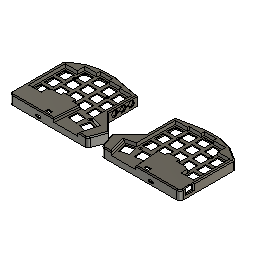
top_3x5_2 (Autodesk Fusion 360 design; units mm, degrees)
Autodesk Fusion 360 part; units mm, degrees
sketch "case_plate_3x5_2" plane through (0, 0, 0) normal (0, 0, 1) x (1, 0, 0)
  line L0 (-131.5, -112.72) -> (-13.7052, -112.72)
  line L1 (-131.5, -30.9488) -> (-131.5, -112.72)
  line L2 (-72.4047, -13.5) -> (-91.6231, -13.5)
  line L3 (-91.6231, -13.5) -> (-111.8983, -18.5688)
  line L4 (-32.5, -21.174) -> (-72.3112, -13.518)
  line L5 (-6.0652, -91.7293) -> (-32.5, -65.3353)
  line L6 (-111.8983, -18.5688) -> (-131.5, -30.9488)
  line L7 (-72.3112, -13.518) -> (-72.4047, -13.5)
  line L8 (-13.7052, -112.72) -> (-6.0652, -91.7293)
  line L9 (-32.5, -65.3353) -> (-32.5, -21.174)
  line L10 (-113.0931, -15.7752) -> (-134.5, -29.2953)
  line L11 (-72.1189, -10.5) -> (-91.9924, -10.5)
  line L12 (-29.5, -64.0913) -> (-29.5, -18.6959)
  line L13 (-11.6046, -115.72) -> (-2.5919, -90.9579)
  line L14 (-134.5, -115.72) -> (-11.6046, -115.72)
  line L15 (-2.5919, -90.9579) -> (-29.5, -64.0913)
  line L16 (-91.9924, -10.5) -> (-113.0931, -15.7752)
  line L17 (-134.5, -29.2953) -> (-134.5, -115.72)
  line L18 (-29.5, -18.6959) -> (-72.1189, -10.5)
  line L19 (-72.2904, -12.3) -> (-91.7708, -12.3)
  line L20 (-132.7, -30.2874) -> (-132.7, -113.92)
  line L21 (-4.6759, -91.4207) -> (-31.3, -64.8377)
  line L22 (-31.3, -20.1828) -> (-72.2904, -12.3)
  line L23 (-132.7, -113.92) -> (-12.865, -113.92)
  line L24 (-12.865, -113.92) -> (-4.6759, -91.4207)
  line L25 (-31.3, -64.8377) -> (-31.3, -20.1828)
  line L26 (-91.7708, -12.3) -> (-112.3762, -17.4513)
  line L27 (-112.3762, -17.4513) -> (-132.7, -30.2874)
  line L28 (-133.3, -29.9567) -> (-133.3, -114.52)
  line L29 (-12.4448, -114.52) -> (-3.9812, -91.2664)
  line L30 (-112.6152, -16.8926) -> (-133.3, -29.9567)
  line L31 (-71.9712, -11.7504) -> (-72.2332, -11.7)
  line L32 (-30.7, -64.5889) -> (-30.7, -19.6872)
  line L33 (-133.3, -114.52) -> (-12.4448, -114.52)
  line L34 (-30.7, -19.6872) -> (-71.9712, -11.7504)
  line L35 (-3.9812, -91.2664) -> (-30.7, -64.5889)
  line L36 (-72.2332, -11.7) -> (-91.8447, -11.7)
  line L37 (-91.8447, -11.7) -> (-112.6152, -16.8926)
  circle A0 centre (-108, -39.5) radius 2.2
  circle A1 centre (-56, -39.5) radius 2.2
  circle A2 centre (-39.8644, -83.3241) radius 2.2
  line L38 (-96.5, -91.61) -> (-129.5, -91.61)
  line L39 (-96.5, -109.61) -> (-96.5, -91.61)
  line L40 (-129.5, -109.61) -> (-96.5, -109.61)
  line L41 (-129.5, -91.61) -> (-129.5, -109.61)
  line L42 (-92.975, -106.99) -> (-92.975, -112.84)
  line L43 (-84.175, -112.84) -> (-84.175, -106.99)
  line L44 (-84.175, -106.99) -> (-92.975, -106.99)
  line L45 (-82.175, -107.975) -> (-82.175, -111.475)
  line L46 (-82.175, -111.475) -> (-73.175, -111.475)
  line L47 (-73.175, -107.975) -> (-82.175, -107.975)
  line L48 (-73.175, -111.475) -> (-73.175, -107.975)
  line L49 (-17.3936, -82.1718) -> (-25.1718, -74.3936)
  line L50 (-25.1718, -74.3936) -> (-31.6064, -80.8282)
  line L51 (-21.0041, -85.7823) -> (-17.3936, -82.1718)
  line L52 (-96.8, -88.45) -> (-96.8, -79.55)
  line L53 (-96.8, -79.55) -> (-105.2875, -79.55)
  line L54 (-105.4, -79.6909) -> (-105.4, -88.45)
  line L55 (-105.4, -88.45) -> (-96.8, -88.45)
  line L56 (-127, -73) -> (-127, -87)
  line L57 (-113, -73) -> (-127, -73)
  line L58 (-113, -87) -> (-113, -73)
  line L59 (-127, -87) -> (-113, -87)
  line L60 (-127, -54) -> (-127, -68)
  line L61 (-113, -68) -> (-113, -54)
  line L62 (-127, -68) -> (-113, -68)
  line L63 (-113, -54) -> (-127, -54)
  line L64 (-113, -35) -> (-127, -35)
  line L65 (-127, -35) -> (-127, -49)
  line L66 (-127, -49) -> (-113, -49)
  line L67 (-113, -49) -> (-113, -35)
  line L68 (-94, -61) -> (-108, -61)
  line L69 (-94, -75) -> (-94, -61)
  line L70 (-108, -61) -> (-108, -75)
  line L71 (-108, -75) -> (-94, -75)
  line L72 (-108, -56) -> (-94, -56)
  line L73 (-94, -56) -> (-94, -42)
  line L74 (-94, -42) -> (-108, -42)
  line L75 (-108, -42) -> (-108, -56)
  line L76 (-94, -37) -> (-94, -23)
  line L77 (-108, -37) -> (-94, -37)
  line L78 (-108, -23) -> (-108, -37)
  line L79 (-94, -23) -> (-108, -23)
  line L80 (-89, -70) -> (-75, -70)
  line L81 (-89, -56) -> (-89, -70)
  line L82 (-75, -56) -> (-89, -56)
  line L83 (-75, -70) -> (-75, -56)
  line L84 (-75, -37) -> (-89, -37)
  line L85 (-89, -37) -> (-89, -51)
  line L86 (-89, -51) -> (-75, -51)
  line L87 (-75, -51) -> (-75, -37)
  line L88 (-89, -32) -> (-75, -32)
  line L89 (-75, -18) -> (-89, -18)
  line L90 (-89, -18) -> (-89, -32)
  line L91 (-75, -32) -> (-75, -18)
  line L92 (-70, -61) -> (-70, -75)
  line L93 (-56, -75) -> (-56, -61)
  line L94 (-70, -75) -> (-56, -75)
  line L95 (-56, -61) -> (-70, -61)
  line L96 (-56, -42) -> (-70, -42)
  line L97 (-70, -42) -> (-70, -56)
  line L98 (-56, -56) -> (-56, -42)
  line L99 (-70, -56) -> (-56, -56)
  line L100 (-70, -23) -> (-70, -37)
  line L101 (-70, -37) -> (-56, -37)
  line L102 (-56, -37) -> (-56, -23)
  line L103 (-56, -23) -> (-70, -23)
  line L104 (-37, -63.5) -> (-51, -63.5)
  line L105 (-51, -77.5) -> (-37, -77.5)
  line L106 (-51, -63.5) -> (-51, -77.5)
  line L107 (-37, -77.5) -> (-37, -63.5)
  line L108 (-51, -58.5) -> (-37, -58.5)
  line L109 (-37, -58.5) -> (-37, -44.5)
  line L110 (-51, -44.5) -> (-51, -58.5)
  line L111 (-37, -44.5) -> (-51, -44.5)
  line L112 (-37, -25.5) -> (-51, -25.5)
  line L113 (-51, -25.5) -> (-51, -39.5)
  line L114 (-51, -39.5) -> (-37, -39.5)
  line L115 (-37, -39.5) -> (-37, -25.5)
  line L116 (-45.8527, -98.8543) -> (-44.6325, -84.9076)
  line L117 (-59.7995, -97.6341) -> (-45.8527, -98.8543)
  line L118 (-58.5793, -83.6874) -> (-59.7995, -97.6341)
  line L119 (-44.6325, -84.9076) -> (-58.5793, -83.6874)
  line L120 (-22.4025, -90.0663) -> (-35.9254, -86.4429)
  line L121 (-39.5489, -99.9658) -> (-26.0259, -103.5893)
  line L122 (-35.9254, -86.4429) -> (-39.5489, -99.9658)
  line L123 (-26.0259, -103.5893) -> (-22.4025, -90.0663)
  line L124 (-131.5, -89.75) -> (-110.25, -89.75)
  line L125 (-110.25, -89.75) -> (-110.25, -79.7)
  line L126 (-129.75, -89.75) -> (-129.75, -32.25)
  line L127 (-110.75, -32.25) -> (-129.75, -32.25)
  line L128 (-91.25, -77.75) -> (-91.25, -72.75)
  line L129 (-91.75, -20.25) -> (-110.75, -20.25)
  line L130 (-110.75, -20.25) -> (-110.75, -32.25)
  line L131 (-91.25, -72.75) -> (-72.75, -72.75)
  line L132 (-72.25, -20.25) -> (-72.25, -15.25)
  line L133 (-72.25, -15.25) -> (-91.75, -15.25)
  line L134 (-91.75, -15.25) -> (-91.75, -20.25)
  line L135 (-72.75, -77.75) -> (-60.8203, -77.75)
  line L136 (-72.75, -72.75) -> (-72.75, -77.75)
  line L137 (-53.25, -22.75) -> (-53.25, -20.25)
  line L138 (-53.25, -20.25) -> (-72.25, -20.25)
  line L139 (-34.25, -65.3353) -> (-34.25, -22.75)
  line L140 (-34.25, -22.75) -> (-53.25, -22.75)
  line L141 (-62.7787, -100.134) -> (-43.1315, -101.8529)
  line L142 (-64.1423, -115.72) -> (-60.8203, -77.75)
  line L143 (-43.1315, -101.8529) -> (-24.0814, -106.9573)
  line L144 (-26.4293, -115.72) -> (-19.0344, -88.1218)
  line L145 (-34.25, -84.0448) -> (-6.2465, -91.5483)
  line L146 (-32.5, -65.3353) -> (-34.25, -65.3353)
  line L147 (-34.25, -84.0448) -> (-34.25, -65.3353)
  arc A3 (-108, -79.7) -> (-105.8143, -77.75) centre (-108, -77.5) ccw
  line L148 (-105.8143, -77.75) -> (-91.25, -77.75)
  line L149 (-108, -79.7) -> (-110.25, -79.7)
  line L150 (-32.5, -82.702) -> (-32.5, -65.3353)
  line L151 (-32.5, -82.702) -> (-8.7266, -89.072)
  line L152 (-31.6064, -80.8282) -> (-28.7198, -83.7149)
  line L153 (-131.5, -90.95) -> (-109.05, -90.95)
  line L154 (-109.05, -90.95) -> (-109.05, -80.9)
  line L155 (-108, -80.9) -> (-109.05, -80.9)
  arc A4 (-108, -80.9) -> (-104.9247, -78.95) centre (-108, -77.5) ccw
  line L156 (-104.9247, -78.95) -> (-90.05, -78.95)
  line L157 (-90.05, -78.95) -> (-90.05, -73.95)
  line L158 (-90.05, -73.95) -> (-73.95, -73.95)
  line L159 (-73.95, -73.95) -> (-73.95, -78.95)
  line L160 (-73.95, -78.95) -> (-62.1299, -78.95)
  line L161 (-65.3468, -115.72) -> (-62.1299, -78.95)
  constraint coincident L14 L161.start
extrude "Extrude1" add sketch "case_plate_3x5_2" against normal blind 7.6 contours L10 L11 L12 L13 L14 L15 L16 L17 L18 L28 L29 L30 L31 L32 L33 L34 L35 L36 L37 L144 L161 | L14 L33 L142 L161 | L14 L33 L142 L144 makes body 1
extrude "Extrude2" add sketch "case_plate_3x5_2" against normal blind 6.8 contours L0 L1 L2 L3 L4 L5 L6 L7 L8 L9 L19 L20 L21 L22 L23 L24 L25 L26 L27 L144 L161 | L0 L23 L142 L161 | L0 L23 L142 L144 | L19 L20 L21 L22 L23 L24 L25 L26 L27 L28 L29 L30 L31 L32 L33 L34 L35 L36 L37 L144 L161 | L23 L33 L142 L161 | L23 L33 L142 L144 bodies 1
extrude "Extrude3" add sketch "case_plate_3x5_2" along normal blind 7 contours L0 L1 L2 L3 L4 L5 L6 L7 L8 L9 L19 L20 L21 L22 L23 L24 L25 L26 L27 L144 L161 | L0 L1 L124 L125 L128 L131 L135 L136 L142 A3 L148 L149 L153 L154 L155 A4 L156 L157 L158 L159 L160 L161 | L1 L2 L3 L4 L6 L7 L9 L124 L126 L127 L129 L130 L132 L133 L134 L137 L138 L139 L140 L146 | L0 L23 L142 L161 | L19 L20 L21 L22 L23 L24 L25 L26 L27 L28 L29 L30 L31 L32 L33 L34 L35 L36 L37 L144 L161 | L23 L33 L142 L161 | L0 L5 L8 L144 L145 | L10 L11 L12 L13 L14 L15 L16 L17 L18 L28 L29 L30 L31 L32 L33 L34 L35 L36 L37 L144 L161 | L14 L33 L142 L161 | L5 L145 L146 L147 L150 L151 bodies 1
extrude "Extrude4" add sketch "case_plate_3x5_2" along normal blind 1.6 from surface at 5.4 contours L0 L1 L42 L43 L44 L52 L53 L54 L55 L153 L154 L155 A4 L156 L157 L158 L159 L160 L161 | L0 L42 L43 L44 | L52 L53 L54 L55 A4 | L5 L49 L50 L51 L150 L151 L152 | L49 L50 L51 L151 L152 | L38 L39 L40 L41 | L45 L46 L47 L48 bodies 1
extrude "Extrude5" add sketch "case_plate_3x5_2" along normal blind 1.6 contours L124 L125 L126 L127 L128 L129 L130 L131 L132 L133 L134 L135 L136 L137 L138 L139 L140 L141 L142 L143 L144 L145 L147 A3 L148 L149 | L0 L141 L142 L143 L144 | L0 L23 L142 L144 | L23 L33 L142 L144 | L14 L33 L142 L144 | A0 | A1 | A2 bodies 1
move_body "Move1" bodies 1 to x (1, 0, 0) y (0, 1, 0) z (0, 0, 1) at (0, 0, -1.6)
hole "Hole1" at (-108, -39.5, 0) at (-108, -77.5, 0) at (-56, -39.5, 0) at (-39.8644, -83.3241, 0) direction (0, 0, -1) diameter 2.4 depth 10 tip angle 118 countersink diameter 4.4 countersink angle 90 bodies 1
sketch "Sketch2" plane through (-134.5, 0, 0) normal (-1, 0, 0) x (0, -1, 0)
  line L0 (29.2953, 5.4) -> (29.2953, -9.2)
  line L1 (29.2953, -9.2) -> (115.72, -9.2)
  line L2 (115.72, -9.2) -> (115.72, 5.4)
  line L3 (115.72, 5.4) -> (29.2953, 5.4)
  line L4 (109.61, 0) -> (91.61, 0)
  line L5 (87.8309, 4.2) -> (115.72, 4.2)
  line L6 (87.7335, -3.8) -> (115.72, -3.8)
  line L7 (94.61, 4.2) -> (94.61, -3.8)
  line L8 (106.61, 4.2) -> (106.61, -3.8)
  dimension "d17" = 1.2
  dimension "d18" = 8
  dimension "d19" = 3
  dimension "d20" = 12
  constraint coincident L2 L5.end
  constraint perpendicular L2 L5
  constraint coincident L2 L6.end
  constraint perpendicular L2 L6
  constraint coincident L5 L7.start
  constraint coincident L6 L7.end
  constraint perpendicular L6 L7
  constraint coincident L5 L8.start
  constraint coincident L6 L8.end
  constraint perpendicular L6 L8
  measures "d17" distance of L3 L5
  measures "d18" distance of L5 L6
  measures "d19" distance of L4.end L7
  measures "d20" distance of L7 L8
extrude "Extrude6" cut sketch "Sketch2" against normal up to surface (3 mm away) contours L4 L5 L7 L8 | L4 L6 L7 L8 bodies 1
chamfer "Chamfer1" distance 1 angle 45 4 edges at (-134.5, -94.61, 0.2) (-134.5, -100.61, -3.8) (-134.5, -106.61, 0.2) (-134.5, -100.61, 4.2) on bodies 1
sketch "Sketch3" plane through (0, -115.72, 0) normal (0, -1, 0) x (1, 0, 0)
  line L0 (-134.5, 5.4) -> (-134.5, -9.2)
  line L1 (-134.5, -9.2) -> (-11.6046, -9.2)
  line L2 (-11.6046, -9.2) -> (-11.6046, 5.4)
  line L3 (-11.6046, 5.4) -> (-26.4293, 5.4)
  line L4 (-26.4293, 5.4) -> (-26.4293, 0)
  line L5 (-26.4293, 0) -> (-64.1423, 0)
  line L6 (-64.1423, 0) -> (-64.1423, 5.4)
  line L7 (-64.1423, 5.4) -> (-134.5, 5.4)
  line L8 (-84.175, 0) -> (-92.975, 0)
  line L9 (-96.2282, -5) -> (-78.2899, -5) construction
  line L10 (-96.4337, -4.25) -> (-77.5367, -4.25) construction
  line L11 (-90.575, 0) -> (-90.575, -4.25) construction
  line L12 (-86.575, 0) -> (-86.575, -4.25) construction
  line L13 (-90.575, -5.75) -> (-86.575, -5.75)
  arc A0 (-86.575, -5.75) -> (-86.575, -2.75) centre (-86.575, -4.25) ccw
  line L14 (-86.575, -2.75) -> (-90.575, -2.75)
  arc A1 (-90.575, -2.75) -> (-90.575, -5.75) centre (-90.575, -4.25) ccw
  line L15 (-90.575, -4.25) -> (-86.575, -4.25) construction
  dimension "d24" = 10.4
  dimension "d25" = 0.75
  dimension "d26" = 2.4
  dimension "d27" = 4
  dimension "d28" = 3
  constraint horizontal L9
  constraint horizontal L10
  constraint coincident L8 L11.start
  constraint coincident L10 L11.end
  constraint perpendicular L10 L11
  constraint coincident L8 L12.start
  constraint coincident L10 L12.end
  constraint perpendicular L10 L12
  constraint tangent L13 A0
  constraint tangent A0 L14
  constraint parallel L13 L14
  constraint tangent L14 A1
  constraint tangent L13 A1
  constraint coincident L12.end A0.centre
  constraint perpendicular L12 L15
  constraint coincident L11.end A1.centre
  measures "d24" distance of L7 L9
  measures "d25" distance of L9 L10
  measures "d26" distance of L8.end L11
  measures "d27" distance of L11 L12
  measures "d28" diameter of A0
extrude "Extrude7" cut sketch "Sketch3" along normal up to surface (-3 mm away) and the other way blind -1 contours L13 A0 L14 A1 bodies 1
sketch "Sketch4" plane through (0, 0, -5.75) normal (0, 0, 1) x (-1, 0, 0)
  line L0 (90.575, 115.72) -> (86.575, 115.72)
  line L1 (86.575, 115.72) -> (86.575, 112.72)
  line L2 (86.575, 112.72) -> (90.575, 112.72)
  line L3 (90.575, 112.72) -> (90.575, 115.72)
  line L4 (90.575, 114.22) -> (86.575, 114.22)
  constraint midpoint L3 L4.start
  constraint midpoint L1 L4.end
extrude "Extrude8" cut sketch "Sketch4" against normal up to surface (2.65 mm away) contours L1 L2 L3 L4 bodies 1
chamfer "Chamfer2" distance 0.5 angle 45 4 edges at (-88.575, -115.72, -2.75) (-85.075, -115.72, -4.25) (-88.575, -115.72, -5.75) (-92.075, -115.72, -4.25) on bodies 1
sketch "Sketch5" plane through (-46.7728, -46.8452, 0) normal (0.70656, 0.707653, 0) x (-0.707653, 0.70656, 0)
  line L0 (-62.433, 5.4) -> (-62.433, -9.2)
  line L1 (-62.433, -9.2) -> (-24.4086, -9.2)
  line L2 (-24.4086, -9.2) -> (-24.4086, 5.4)
  line L3 (-24.4086, 5.4) -> (-62.433, 5.4)
  line L4 (-62.433, -5) -> (-24.4086, -5) construction
  line L5 (-45.7507, 0) -> (-34.7507, 0)
  line L6 (-48.9332, -4.5) -> (-31.4162, -4.5)
  line L7 (-48.8433, -5.5) -> (-31.4162, -5.5)
  line L8 (-43.7507, -4.5) -> (-43.7507, -5.5)
  line L9 (-36.7507, -4.5) -> (-36.7507, -5.5)
  dimension "d36" = 10.4
  dimension "d37" = 0.5
  dimension "d38" = 0.5
  dimension "d39" = 2
  dimension "d40" = 7
  constraint coincident L0 L4.start
  constraint coincident L2 L4.end
  constraint perpendicular L2 L4
  constraint horizontal L6
  constraint perpendicular L2 L7
  constraint coincident L6 L8.start
  constraint coincident L7 L8.end
  constraint perpendicular L7 L8
  constraint coincident L6 L9.start
  constraint coincident L7 L9.end
  constraint perpendicular L7 L9
  measures "d36" distance of L3 L4
  measures "d37" distance of L4 L6
  measures "d38" distance of L4 L7
  measures "d39" distance of L5.start L8
  measures "d40" distance of L8 L9
extrude "Extrude9" cut sketch "Sketch5" against normal up to surface (3 mm away) contours L6 L7 L8 L9 bodies 1
sketch "Sketch6" plane through (0, 0, 5.4) normal (0, 0, 1) x (-1, 0, 0)
  arc A0 (108, 79.7) -> (105.8143, 77.75) centre (108, 77.5) ccw
  line L0 (108, 79.7) -> (110.25, 79.7)
  line L1 (110.25, 79.7) -> (110.25, 89.75)
  line L2 (110.25, 89.75) -> (129.75, 89.75)
  line L3 (129.75, 89.75) -> (129.75, 32.25)
  line L4 (129.75, 32.25) -> (110.75, 32.25)
  line L5 (110.75, 32.25) -> (110.75, 20.25)
  line L6 (110.75, 20.25) -> (91.75, 20.25)
  line L7 (91.75, 20.25) -> (91.75, 15.25)
  line L8 (91.75, 15.25) -> (72.25, 15.25)
  line L9 (72.25, 15.25) -> (72.25, 20.25)
  line L10 (72.25, 20.25) -> (53.25, 20.25)
  line L11 (53.25, 20.25) -> (53.25, 22.75)
  line L12 (53.25, 22.75) -> (34.25, 22.75)
  line L13 (34.25, 22.75) -> (34.25, 84.0448)
  line L14 (34.25, 84.0448) -> (19.0344, 88.1218)
  line L15 (19.0344, 88.1218) -> (26.4293, 115.72)
  line L16 (26.4293, 115.72) -> (11.6046, 115.72)
  line L17 (11.6046, 115.72) -> (2.5919, 90.9579)
  line L18 (2.5919, 90.9579) -> (29.5, 64.0913)
  line L19 (29.5, 64.0913) -> (29.5, 18.6959)
  line L20 (29.5, 18.6959) -> (72.1189, 10.5)
  line L21 (72.1189, 10.5) -> (91.9924, 10.5)
  line L22 (91.9924, 10.5) -> (113.0931, 15.7752)
  line L23 (113.0931, 15.7752) -> (134.5, 29.2953)
  line L24 (134.5, 29.2953) -> (134.5, 115.72)
  line L25 (134.5, 115.72) -> (64.1423, 115.72)
  line L26 (64.1423, 115.72) -> (60.8203, 77.75)
  line L27 (60.8203, 77.75) -> (72.75, 77.75)
  line L28 (72.75, 77.75) -> (72.75, 72.75)
  line L29 (72.75, 72.75) -> (91.25, 72.75)
  line L30 (91.25, 72.75) -> (91.25, 77.75)
  line L31 (91.25, 77.75) -> (105.8143, 77.75)
  line L32 (73.175, 107.975) -> (82.175, 107.975)
  line L33 (82.175, 107.975) -> (82.175, 111.475)
  line L34 (82.175, 111.475) -> (73.175, 111.475)
  line L35 (73.175, 111.475) -> (73.175, 107.975)
  line L36 (80.675, 107.975) -> (80.675, 111.475)
  line L37 (74.675, 107.975) -> (74.675, 111.475)
  point P0 (82.175, 107.975)
  dimension "d43" = 1.5
  dimension "d44" = 6
  constraint coincident L32 L36.start
  constraint coincident L34 L36.end
  constraint perpendicular L34 L36
  constraint coincident L32 L37.start
  constraint coincident L34 L37.end
  constraint perpendicular L34 L37
  measures "d43" distance of L36 P0
  measures "d44" distance of L36 L37
extrude "Extrude10" cut sketch "Sketch6" against normal up to surface (1.6 mm away) contours L32 L34 L36 L37 bodies 1
chamfer "Chamfer3" distance 0.4 angle 45 4 edges at (-77.675, -107.975, 5.4) (-80.675, -109.725, 5.4) (-77.675, -111.475, 5.4) (-74.675, -109.725, 5.4) on bodies 1
sketch "Sketch7" plane through (-29.5, 0, 0) normal (1, 0, 0) x (0, 1, 0)
  line L0 (-64.0913, 5.4) -> (-64.0913, -9.2)
  line L1 (-64.0913, -9.2) -> (-18.6959, -9.2)
  line L2 (-18.6959, -9.2) -> (-18.6959, 5.4)
  line L3 (-18.6959, 5.4) -> (-64.0913, 5.4)
  line L4 (-64.0913, -1.5) -> (-18.6959, -1.5) construction
  line L5 (-52.0795, 2.4639) -> (-56.6694, 2.486)
  line L6 (-56.6694, 2.486) -> (-58.9835, -1.4778)
  line L7 (-58.9835, -1.4778) -> (-56.7078, -5.4639)
  line L8 (-56.7078, -5.4639) -> (-52.1179, -5.486)
  line L9 (-52.1179, -5.486) -> (-49.8038, -1.5222)
  line L10 (-49.8038, -1.5222) -> (-52.0795, 2.4639)
  line L11 (-39.0795, 2.4639) -> (-43.6694, 2.486)
  line L12 (-43.6694, 2.486) -> (-45.9835, -1.4778)
  line L13 (-45.9835, -1.4778) -> (-43.7078, -5.4639)
  line L14 (-43.7078, -5.4639) -> (-39.1179, -5.486)
  line L15 (-39.1179, -5.486) -> (-36.8038, -1.5222)
  line L16 (-36.8038, -1.5222) -> (-39.0795, 2.4639)
  line L17 (-26.0795, 2.4639) -> (-30.6694, 2.486)
  line L18 (-30.6694, 2.486) -> (-32.9835, -1.4778)
  line L19 (-32.9835, -1.4778) -> (-30.7078, -5.4639)
  line L20 (-30.7078, -5.4639) -> (-26.1179, -5.486)
  line L21 (-26.1179, -5.486) -> (-23.8038, -1.5222)
  line L22 (-23.8038, -1.5222) -> (-26.0795, 2.4639)
  line L23 (-54.3936, -2.25) -> (-28.3936, -2.25)
  arc A0 (-28.3936, -2.25) -> (-28.3936, -0.75) centre (-28.3936, -1.5) ccw
  line L24 (-28.3936, -0.75) -> (-54.3936, -0.75)
  arc A1 (-54.3936, -0.75) -> (-54.3936, -2.25) centre (-54.3936, -1.5) ccw
  line L25 (-54.3936, -1.5) -> (-28.3936, -1.5) construction
  point P0 (-41.3936, -1.5)
  point P1 (-28.3936, -1.5)
  point P2 (-54.3936, -1.5)
  point P3 (-54.3936, -1.5)
  point P4 (-41.3936, -1.5)
  point P5 (-28.3936, -1.5)
  dimension "d48" = 6.9
  dimension "d49" = 13
  dimension "d50" = 13
  dimension "d51" = 3.975
  dimension "d52" = 3.975
  dimension "d53" = 3.975
  dimension "d54" = 1.5
  constraint coincident L0 L4.start
  constraint coincident L2 L4.end
  constraint perpendicular L2 L4
  constraint midpoint L4 P4
  constraint coincident L4 P5
  constraint coincident L4 P3
  constraint coincident P3 P2
  constraint coincident P4 P0
  constraint coincident P5 P1
  constraint tangent L23 A0
  constraint tangent A0 L24
  constraint parallel L23 L24
  constraint tangent L24 A1
  constraint tangent L23 A1
  constraint parallel L4 L25
  measures "d48" distance of L3 L4
  measures "d49" distance of P4 P3
  measures "d50" distance of P4 P5
  measures "d51" distance of P3 L10
  measures "d52" distance of P4 L16
  measures "d53" distance of P5 L22
  measures "d54" diameter of A0
extrude "Extrude11" cut sketch "Sketch7" against normal blind 2 contours L5 L6 L7 L8 L9 L10 L23 L24 A1 | L9 L10 L12 L13 L23 L24 | L9 L10 L23 L24 A1 | L12 L13 L15 L16 L23 L24 | L11 L12 L16 L24 | L15 L16 L18 L19 L23 L24 | L13 L14 L15 L23 | L18 L19 L23 A0 L24 | L17 L18 L19 L20 L21 L22 L23 A0 L24 bodies 1
chamfer "Chamfer4" distance 0.4 angle 45 18 edges at (-29.5, -24.9416, 0.4709) (-29.5, -24.9608, -3.5041) (-29.5, -28.4128, -5.475) (-29.5, -31.6252, -3.8569) (-29.5, -28.3744, 2.475) (-29.5, -31.614, 0.868) (-29.5, -38.1621, 0.8569) (-29.5, -38.1733, -3.868) (-29.5, -41.4128, -5.475) (-29.5, -44.6252, -3.8569) (-29.5, -41.3744, 2.475) (-29.5, -44.614, 0.868) (-29.5, -51.1621, 0.8569) (-29.5, -51.1733, -3.868) (-29.5, -54.4128, -5.475) (-29.5, -57.8456, -3.4709) (-29.5, -54.3744, 2.475) (-29.5, -57.8265, 0.5041) on bodies 1
sketch "Sketch8" plane through (-46.7728, -46.8452, 0) normal (0.70656, 0.707653, 0) x (-0.707653, 0.70656, 0)
  line L0 (-43.7507, -4.5) -> (-36.7507, -4.5)
  line L1 (-36.7507, -4.5) -> (-36.7507, -5.5)
  line L2 (-36.7507, -5.5) -> (-43.7507, -5.5)
  line L3 (-43.7507, -5.5) -> (-43.7507, -4.5)
  line L4 (-62.433, 5.4) -> (-62.433, -9.2)
  line L5 (-62.433, -9.2) -> (-24.4086, -9.2)
  line L6 (-24.4086, -9.2) -> (-24.4086, 5.4)
  line L7 (-24.4086, 5.4) -> (-62.433, 5.4)
  line L8 (-62.433, -1.5) -> (-24.4086, -1.5) construction
  line L9 (-48.1317, 2.4713) -> (-52.7217, 2.4786)
  line L10 (-52.7217, 2.4786) -> (-55.023, -1.4927)
  line L11 (-55.023, -1.4927) -> (-52.7343, -5.4713)
  line L12 (-52.7343, -5.4713) -> (-48.1444, -5.4786)
  line L13 (-48.1444, -5.4786) -> (-45.8431, -1.5073)
  line L14 (-45.8431, -1.5073) -> (-48.1317, 2.4713)
  line L15 (-36.9986, -1.5073) -> (-34.6973, -5.4786)
  line L16 (-34.6973, -5.4786) -> (-30.1073, -5.4713)
  line L17 (-30.1073, -5.4713) -> (-27.8187, -1.4927)
  line L18 (-27.8187, -1.4927) -> (-30.12, 2.4786)
  line L19 (-30.12, 2.4786) -> (-34.7099, 2.4713)
  line L20 (-34.7099, 2.4713) -> (-36.9986, -1.5073)
  line L21 (-50.433, -2.25) -> (-32.4086, -2.25)
  arc A0 (-32.4086, -2.25) -> (-32.4086, -0.75) centre (-32.4086, -1.5) ccw
  line L22 (-32.4086, -0.75) -> (-50.433, -0.75)
  arc A1 (-50.433, -0.75) -> (-50.433, -2.25) centre (-50.433, -1.5) ccw
  line L23 (-50.433, -1.5) -> (-32.4086, -1.5) construction
  point P0 (-50.433, -1.5)
  point P1 (-32.4086, -1.5)
  point P2 (-50.433, -1.5)
  point P3 (-32.4086, -1.5)
  dimension "d58" = 6.9
  dimension "d59" = 8
  dimension "d60" = 12
  dimension "d61" = 3.975
  dimension "d62" = 3.975
  dimension "d63" = 1.5
  constraint coincident L4 L8.start
  constraint coincident L6 L8.end
  constraint perpendicular L6 L8
  constraint coincident L8 P2
  constraint coincident L8 P3
  constraint coincident P2 P0
  constraint coincident P3 P1
  constraint tangent L21 A0
  constraint tangent A0 L22
  constraint parallel L21 L22
  constraint tangent L22 A1
  constraint tangent L21 A1
  constraint parallel L8 L23
  measures "d58" distance of L7 L8
  measures "d59" distance of L6 P3
  measures "d60" distance of L4 P2
  measures "d61" distance of P2 L14
  measures "d62" distance of P3 L20
  measures "d63" diameter of A0
extrude "Extrude12" cut sketch "Sketch8" against normal blind 2 contours L9 L10 L11 L12 L13 L14 L21 L22 A1 | L13 L14 L15 L20 L21 L22 | L13 L14 L21 L22 A1 | L15 L20 L21 A0 L22 | L15 L16 L17 L18 L19 L20 L21 A0 L22 bodies 1
chamfer "Chamfer5" distance 0.4 angle 45 12 edges at (-8.6499, -84.9092, 0.493) (-8.6455, -84.9137, -3.482) (-11.0793, -82.4836, -5.475) (-13.3653, -80.2011, -3.8643) (-13.3679, -80.1985, 0.8607) (-11.0882, -82.4747, 2.475) (-21.5546, -72.0244, 0.8607) (-23.8343, -69.7483, 2.475) (-26.2726, -67.3138, 0.493) (-26.2771, -67.3093, -3.482) (-23.8432, -69.7393, -5.475) (-21.5572, -72.0218, -3.8643) on bodies 1
fillet "Fillet1" radius 5 6 edges at (-11.6046, -115.72, -1.9) (-134.5, -115.72, -1.9) (-134.5, -29.2953, -1.9) (-113.0931, -15.7752, -1.9) (-91.9924, -10.5, -1.9) (-72.1189, -10.5, -1.9) on bodies 1
fillet "Fillet1" radius 5 6 edges at (-133.3, -114.52, -8.8) (-133.3, -29.9567, -8.8) (-112.6152, -16.8926, -8.8) (-91.8447, -11.7, -8.8) (-72.2332, -11.7, -8.8) (-12.4448, -114.52, -8.8) on bodies 1
fillet "Fillet1" radius 2 6 edges at (-13.7052, -112.72, -5) (-131.5, -112.72, -2.3) (-131.5, -30.9488, -5) (-111.8983, -18.5688, -5) (-91.6231, -13.5, -5) (-72.4047, -13.5, -5) on bodies 1
chamfer "Chamfer6" distance 1.5 angle 45 18 edges at (-22.7319, -101.9209, 5.4) (-20.7675, -115.72, 5.4) (-12.2377, -114.8157, 5.4) (-6.4995, -101.694, 5.4) (-16.046, -77.5246, 5.4) (-29.5, -41.3936, 5.4) (-50.5755, -14.643, 5.4) (-72.121, -10.5225, 5.4) (-81.9861, -10.5, 5.4) (-91.9878, -10.5375, 5.4) (-102.452, -13.1149, 5.4) (-113.0679, -15.834, 5.4) (-122.9708, -22.0137, 5.4) (-133.8789, -29.6376, 5.4) (-134.5, -71.3856, 5.4) (-133.0355, -114.2555, 5.4) (-96.8211, -115.72, 5.4) (-62.4813, -96.735, 5.4) on bodies 1
mirror "Mirror1" about plane through (0, 0, 0) normal (1, 0, 0) of bodies 1 makes body 2
